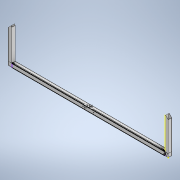
# Autodesk Inventor part: Base_Fundo_Suporte_Lamina
Saved by Autodesk Inventor 2020.4 (Build 244396000, 396)
## iProperties
Created: 2021-05-07
Part Number: Base_Fundo_Suporte_Lamina
Material: Genérico
Document SubType Name: Modeling
Designer: Alison
Density: 1 g/cm^3
Appearance: Padrão
Author: Alison
Autodesk Inventor part; units mm, degrees
ref_plane "YZ Plane" through (0, 0, 0) normal (1, 0, 0) x (0, 1, 0)
ref_plane "XZ Plane" through (0, 0, 0) normal (0, 1, 0) x (-1, 0, 0)
ref_plane "XY Plane" through (0, 0, 0) normal (0, 0, 1) x (1, 0, 0)
sketch "Esboço1" plane through (0, 0, 0) normal (0, 1, 0) x (-1, 0, 0)
  line L0 (0, 0) -> (40, 0)
  line L1 (40, 0) -> (40, -40)
  line L2 (40, -40) -> (0, -40)
  line L3 (0, -40) -> (0, 0)
  line L4 (0, 0) -> (1.5, 0)
  line L5 (1.5283, -1.4997) -> (38.5283, -1.4997)
  line L6 (38.5283, -1.4997) -> (38.5283, -38.4997)
  line L7 (38.5283, -38.4997) -> (1.5283, -38.4997)
  line L8 (1.5283, -38.4997) -> (1.5283, -1.4997)
  line L9 (1804, 0) -> (1764, 0)
  line L10 (1764, 0) -> (1764, -40)
  line L11 (1764, -40) -> (1804, -40)
  line L12 (1804, -40) -> (1804, 0)
  line L13 (1804, 0) -> (1802.5, 0)
  line L14 (1804, -1.4997) -> (1804, 0)
  line L15 (1802.5, -1.4997) -> (1765.5, -1.4997)
  line L16 (1765.5, -1.4997) -> (1765.5, -38.4997)
  line L17 (1765.5, -38.4997) -> (1802.5, -38.4997)
  line L18 (1802.5, -38.4997) -> (1802.5, -1.4997)
  line L19 (38.5283, -1.4997) -> (1.5283, -1.4997)
  line L20 (1.5283, -1.4997) -> (1.5283, -38.4997)
  line L21 (1.5283, -38.4997) -> (38.5283, -38.4997)
  line L22 (38.5283, -38.4997) -> (38.5283, -1.4997)
  dimension "d0" = 40
  dimension "d1" = 40
  dimension "d2" = 1.5
  dimension "d3" = 1.5
  dimension "d4" = 37
  dimension "d5" = 37
  dimension "d6" = 1804
  dimension "d8" = 40
  dimension "d9" = 40
  dimension "d10" = 1.5
  dimension "d11" = 37
  dimension "d12" = 37
  dimension "d15" = 37
  dimension "d16" = 37
  constraints: 46 end point, 10 parallel, 6 horizontal, 5 perpendicular, 1 point on line
  measures "d0" distance of L1.end L2.end
  measures "d1" distance of L0.end L1.end
  measures "d2" distance of L0.start L4.end
  measures "d3" distance of L4.end L5.start
  measures "d4" distance of L6.end L7.end
  measures "d5" distance of L5.end L6.end
  measures "d6" distance of L0.start L9.start
  measures "d8" distance of L11.end L10.end
  measures "d9" distance of L10.end L9.end
  measures "d10" distance of L14.start L15.start
  measures "d11" distance of L17.end L16.end
  measures "d12" distance of L16.end L15.end
  measures "d15" distance of L21.end L7.end
  measures "d16" distance of L7.end L19.end
extrude "Extrusão1" add sketch "Esboço1" along normal blind 400
sketch "Esboço2" plane through (0, 0, 0) normal (0, 1, 0) x (-1, 0, 0)
  line L0 (38.4659, -1.6068) -> (1.4659, -1.6068)
  line L1 (1.4659, -1.6068) -> (1.4659, -38.6068)
  line L2 (1.4659, -38.6068) -> (38.4659, -38.6068)
  line L3 (38.4659, -38.6068) -> (38.4659, -1.6068)
  point P0 (0, 0)
  dimension "d17" = 37
  dimension "d18" = 37
  constraints: 8 end point, 2 parallel, 1 horizontal, 1 perpendicular
  measures "d17" distance of L2.end L1.end
  measures "d18" distance of L1.end L0.end
extrude "Extrusão2" add sketch "Esboço2" along normal blind 1.5
sketch "Esboço3" plane through (0, 0, 0) normal (0, 1, 0) x (-1, 0, 0)
  line L0 (1802.5, -38.4997) -> (1765.5, -38.4997) projected
  line L1 (1765.5, -38.4997) -> (1765.5, -1.4997) projected
  line L2 (1802.5, -38.4997) -> (1765.5, -38.4997)
  line L3 (1765.5, -38.4997) -> (1765.5, -1.4997)
  line L4 (1765.5, -1.4997) -> (1802.5, -1.4997)
  line L5 (1802.5, -1.4997) -> (1802.5, -38.4997)
  point P0 (0, 0)
  constraints: 8 end point, 2 parallel, 1 horizontal, 1 perpendicular
extrude "Extrusão3" add sketch "Esboço3" along normal blind 1.5
sketch "Esboço4" plane through (0, 0, 0) normal (0, 0, 1) x (1, 0, 0)
  line L0 (-40, 0) -> (-40, 400) projected
  line L1 (-40, 0) -> (-1764, 0)
  line L2 (-1764, 0) -> (-1764, 44.8822)
  line L3 (-40, 44.8822) -> (-40, 0)
  line L4 (-1764, 0) -> (-40, 0)
  line L5 (-40, 0) -> (-40, 40)
  line L6 (-40, 40) -> (-1764, 40)
  line L7 (-1764, 40) -> (-1764, 0)
  point P0 (0, 0)
  dimension "d23" = 1724
  dimension "d24" = 1724
  dimension "d25" = 40
  constraints: 14 end point, 3 parallel, 2 horizontal, 2 perpendicular
  measures "d23" distance of L2.end L3.start
  measures "d24" distance of L6.end L5.end
  measures "d25" distance of L5.end L4.end
sketch "Esboço7" plane through (0, 0, 0) normal (1, 0, 0) x (0, 1, 0)
  line L0 (0, 0) -> (1.5, 0)
  line L1 (1.5, 0) -> (1.5, -1.5)
  line L2 (1.5, -1.5) -> (0, -1.5)
  line L3 (0, -1.5) -> (0, 0)
  line L4 (1.5, -1.4997) -> (400, -1.4997) projected
  line L5 (1.5, -1.4997) -> (38.5, -1.4997)
  line L6 (38.5, -1.4997) -> (38.5, -38.4997)
  line L7 (38.5, -38.4997) -> (1.5, -38.4997)
  line L8 (1.5, -38.4997) -> (1.5, -1.4997)
  line L9 (0, 0) -> (400, 0) projected
  line L10 (0, 0) -> (40, 0)
  line L11 (40, 0) -> (40, -40)
  line L12 (40, -40) -> (0, -40)
  line L13 (0, -40) -> (0, 0)
  dimension "d44" = 1.5
  dimension "d45" = 1.5
  dimension "d46" = 37
  dimension "d47" = 37
  dimension "d48" = 40
  dimension "d49" = 40
  constraints: 24 end point, 6 parallel, 3 horizontal, 3 perpendicular
  measures "d44" distance of L1.end L2.end
  measures "d45" distance of L0.end L1.end
  measures "d46" distance of L6.end L7.end
  measures "d47" distance of L5.end L6.end
  measures "d48" distance of L11.end L12.end
  measures "d49" distance of L10.end L11.end
extrude "Extrusão6" add sketch "Esboço7" against normal blind 1804 contours L0 L1 L2 L3 | L9 L11 L4 L1 | L2 L8 L7 L6 L4 L11 L12 L13
sketch "Esboço9" plane through (0, 0, -40) normal (0, 0, -1) x (-1, 0, 0)
  line L0 (40, 40) -> (1764, 40) projected
  line L1 (0, 0) -> (0, 400) projected
  point P0 (842, 20)
  point P1 (962, 20)
  point P2 (0, 373)
  dimension "d87" = 20
  dimension "d88" = 20
  dimension "d89" = 120
  dimension "d90" = 842
  measures "d87" distance from line of L0 point (842, 20)
  measures "d88" distance from line of L0 point (962, 20)
  measures "d89" distance of point (962, 20) point (842, 20)
  measures "d90" distance from line of L1 point (842, 20)
hole "Furo2" at (-842, 20, -40) at (-962, 20, -40) direction (0, 0, 1) diameter 10 depth 200
sketch "Esboço10" plane through (-1764, 40, -40) normal (0, 1, 0) x (1, 0, 0)
  line L0 (1764, -40) -> (1764, 0) projected
  line L1 (1724, -40) -> (0, -40) projected
  point P0 (862, -20)
  dimension "d98" = 902
  dimension "d99" = 20
  measures "d98" distance from line of L0 point (862, -20)
  measures "d99" distance from line of L1 point (862, -20)
hole "Furo3" at (-902, 40, -20) direction (0, -1, 0) diameter 10 depth 200
chamfer "Chanfro8" distance 30 angle 45 1 edges at (0, 400, -20)
chamfer "Chanfro9" distance 10 angle 45 1 edges at (-40, 400, -20)
chamfer "Chanfro10" distance 10 angle 45 1 edges at (-1764, 400, -20)
chamfer "Chanfro11" distance 30 angle 45 1 edges at (-1804, 400, -20)
